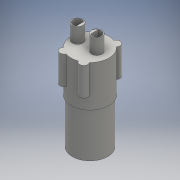
# Autodesk Inventor part: pump
Saved by Autodesk Inventor 2016 (Build 200138000, 138)
## iProperties
Created: 2016-12-04
Part Number: pump
Material: Generic
Document SubType Name: Modeling
Designer: gavri
Density: 1 g/cm^3
Appearance: Default
Author: gavri
Autodesk Inventor part; units mm, degrees
ref_plane "YZ Plane" through (0, 0, 0) normal (1, 0, 0) x (0, 1, 0)
ref_plane "XZ Plane" through (0, 0, 0) normal (0, 1, 0) x (-1, 0, 0)
ref_plane "XY Plane" through (0, 0, 0) normal (0, 0, 1) x (1, 0, 0)
sketch "Sketch1" plane through (0, 0, 0) normal (0, 0, 1) x (1, 0, 0)
  circle A0 centre (0, 0) radius 16
  dimension "d0" = 32
  constraints: 1 centre point, 1 coincident
  measures "d0" diameter of A0
extrude "Extrusion1" add sketch "Sketch1" against normal blind 35
sketch "Sketch2" plane through (0, 0, -35) normal (0, 0, -1) x (-1, 0, 0)
  circle A0 centre (0, 0) radius 15
  dimension "d3" = 30
  constraints: 1 centre point, 1 coincident
  measures "d3" diameter of A0
extrude "Extrusion2" add sketch "Sketch2" along normal blind 38
sketch "Sketch3" plane through (0, 0, -73) normal (0, 0, -1) x (-1, 0, 0)
  circle A0 centre (0, 0) radius 4.064
  constraints: 1 centre point, 1 coincident
extrude "Extrusion3" add sketch "Sketch3" along normal blind 3
sketch "Sketch4" plane through (0, 0, 0) normal (0, 0, 1) x (1, 0, 0)
  point P0 (0, 0)
sketch "Sketch5" plane through (0, 0, 0) normal (0, 0, 1) x (1, 0, 0)
  circle A0 centre (-10.5, 0) radius 4.5
  circle A1 centre (0, 0) radius 15 projected
  circle A2 centre (5.7991, 0) radius 4.5
  dimension "d8" = 9
  constraints: 2 centre point, 1 tangent
  measures "d8" diameter of A0
extrude "Extrusion4" add sketch "Sketch5" along normal blind 13 contours A0 | A2
sketch "Sketch6" plane through (-10.5, 0, 13) normal (0, 0, 1) x (1, 0, 0)
  arc A0 (2.1608, 3.1628) -> (2.1608, -3.1628) centre (0, 0) ccw
  circle A1 centre (16.2991, 0) radius 4.5 projected
  arc A2 (14.1383, -3.1628) -> (14.1383, 3.1628) centre (16.2991, 0) ccw
  circle A3 centre (0, 0) radius 4.5 projected
  line L0 (14.1383, 3.1628) -> (14.1383, -3.1628)
  line L1 (2.1608, 3.1628) -> (2.1608, -3.1628)
  point P0 (10.5, 0)
  constraints: 4 end point, 4 point on circle, 2 centre point, 2 concentric, 1 vertical
extrude "Extrusion5" cut sketch "Sketch6" against normal blind 13 contours L1 A0 | L0 A2
sketch "Sketch7" plane through (0, 0, 0) normal (0, 0, 1) x (1, 0, 0)
  circle A0 centre (0, 0) radius 16 projected
  circle A1 centre (-8.3308, 13.6601) radius 3.5
  line L0 (0, -22.632) -> (0, 23.7921) projected
  circle A2 centre (8.3308, 13.6601) radius 3.5
  line L1 (-22.4, 0) -> (22.4, 0) projected
  circle A3 centre (-8.3308, -13.6601) radius 3.5
  circle A4 centre (8.3308, -13.6601) radius 3.5
  dimension "d14" = 7
  constraints: 4 centre point, 3 symmetric about line, 5 other
  measures "d14" diameter of A1
extrude "Extrusion6" add sketch "Sketch7" against normal blind 24 contours A2 A0 | A0 A2 | A4 A0 | A0 A4 | A3 A0 | A0 A3 | A1 A0 | A0 A1
body "Solid1"
